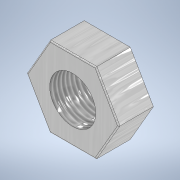
# Autodesk Inventor part: Porca
Saved by Autodesk Inventor 2021 (Build 250183000, 183)
## iProperties
Created: 2021-04-08
Part Number: Porca
Material: Genérico
Document SubType Name: Modeling
Designer: rubia
Density: 1 g/cm^3
Appearance: Polido escovado
Author: rubia
Autodesk Inventor part; units mm, degrees
ref_plane "YZ Plane" through (0, 0, 0) normal (1, 0, 0) x (0, 1, 0)
ref_plane "XZ Plane" through (0, 0, 0) normal (0, 1, 0) x (-1, 0, 0)
ref_plane "XY Plane" through (0, 0, 0) normal (0, 0, 1) x (1, 0, 0)
sketch "Esboço1" plane through (0, 0, 0) normal (0, 0, 1) x (1, 0, 0)
  line L0 (-4, 6.9282) -> (4, 6.9282)
  line L1 (4, 6.9282) -> (8, 0)
  line L2 (8, 0) -> (4, -6.9282)
  line L3 (4, -6.9282) -> (-4, -6.9282)
  line L4 (-4, -6.9282) -> (-8, 0)
  line L5 (-8, 0) -> (-4, 6.9282)
  circle A0 centre (0, 0) radius 4
  dimension "d0" = 8
  dimension "d1" = 8
  constraints: 12 end point, 2 coincident, 1 centre point, 1 horizontal, 13 other
  measures "d0" distance of L0.start L0.end
  measures "d1" diameter of A0
extrude "Extrusão1" add sketch "Esboço1" along normal blind 6
fillet "Arredondamento1" radius 0.2 6 edges at (0, 6.9282, 6) (6, 3.4641, 6) (6, -3.4641, 6) (0, -6.9282, 6) (-6, -3.4641, 6) (-6, 3.4641, 6)
thread "Rosca1" size "M8x0.75" class "6H" standard "ANSI Metric M Profile" length 7
